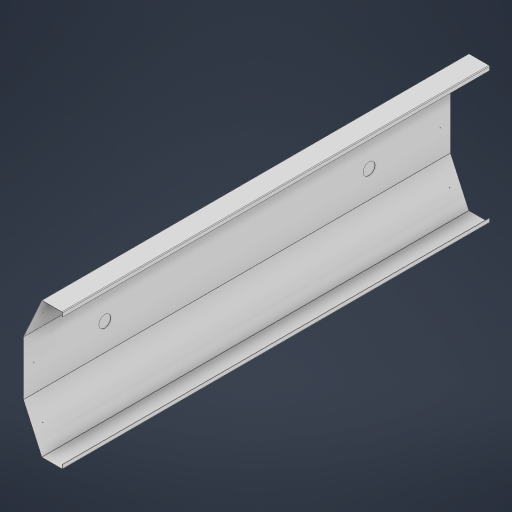
# Autodesk Inventor part: Carcasa
Saved by Autodesk Inventor 2024 (Build 280153000, 153)
## iProperties
Created: 2023-04-23
Part Number: Carcasa
Material: Genérico
Document SubType Name: Sheet Metal
Designer: javie
Density: 1 g/cm^3
Sheet Metal Rule: Por defecto_mm
Appearance: Valor por defecto
Author: javie
Autodesk Inventor part; units mm, degrees
note: some values were not read from the file. Chosen so that the rebuilt part matches the saved one: flange form of "Placa1".
ref_plane "YZ Plane" through (0, 0, 0) normal (1, 0, 0) x (0, 1, 0)
ref_plane "XZ Plane" through (0, 0, 0) normal (0, 1, 0) x (-1, 0, 0)
ref_plane "XY Plane" through (0, 0, 0) normal (0, 0, 1) x (1, 0, 0)
sketch "Boceto1" plane through (0, 0, 0) normal (0, 0, 1) x (1, 0, 0)
  line L0 (-10, 6.5506) -> (-10, 58.1012)
  line L1 (-10, 58.1012) -> (17.1565, 118.1012)
  line L2 (17.1565, 118.1012) -> (47.1565, 118.1012)
  line L3 (47.1565, 118.1012) -> (47.1565, 112.4113)
  line L4 (-10, 6.5506) -> (-10, -21.8988)
  line L5 (-10, -21.8988) -> (17.1565, -81.8988)
  line L6 (17.1565, -81.8988) -> (47.1565, -81.8988)
  line L7 (47.1565, -81.8988) -> (47.1565, -76.2089)
  point P0 (47.1565, 115.2562)
  dimension "d22" = 60
  dimension "d23" = 60
  dimension "d24" = 30
  dimension "d25" = 30
  dimension "d26" = 200
  dimension "d44" = 57.1565
  measures "d22" vertical distance of L0.end L1.end
  measures "d23" vertical distance of L5.start L6.start
  measures "d24" distance of L1.end L2.end
  measures "d25" distance of L6.start L7.start
  measures "d26" distance of L7.start L2.end
  measures "d44" distance from line of L0 point (47.156, 115.256)
contour flange "Pestaña de contorno1" sketch "Boceto1" thickness 0.5 bend radius 0.5 width 629.96 along (0, 0, 1) mid plane no both sides no wall seen from (47.1565, 115.2562, 0) lies toward (1, 0, 0) curves L3 L2 L1 L0 L4 L5 L6 L7
bend "Doblez1"
corner "Esquina1"
sketch "Boceto2" plane through (-10, -21.7909, 629.96) normal (1, 0, 0) x (0, 0, -1)
  circle A0 centre (614.96, 39.8921) radius 0.5
  line L0 (629.96, 79.7842) -> (629.96, 0) projected
  circle A1 centre (15, 39.8921) radius 0.5
  line L1 (0, 0) -> (0, 79.7842) projected
  circle A2 centre (120, 39.8921) radius 9
  circle A3 centre (509.96, 39.8921) radius 9
  point P0 (629.96, 21.7909)
  point P1 (0, 39.8921)
  point P2 (629.96, 39.8921)
  dimension "d16" = 1
  dimension "d17" = 15
  dimension "d18" = 1
  dimension "d19" = 15
  dimension "d27" = 0
  dimension "d40" = 18
  dimension "d41" = 18
  dimension "d42" = 120
  dimension "d43" = 120
  constraints: 4 centre point, 2 midpoint
  measures "d16" diameter of A0
  measures "d17" distance from line of L0 A0.centre
  measures "d18" diameter of A1
  measures "d19" distance of point (0, 39.892) A1.centre
  measures "d27" vertical distance of point (629.96, 39.892) A0.centre
  measures "d40" diameter of A2
  measures "d41" diameter of A3
  measures "d42" distance from line of L1 A2.centre
  measures "d43" distance from line of L0 A3.centre
extrude "Extrusión1" cut sketch "Boceto2" against normal blind 10
sketch "Boceto3" plane through (-9.9555, 58.1995, 629.96) normal (0.9110302, -0.4123397, 0) x (0, 0, -1)
  circle A0 centre (15, 32.7145) radius 0.5
  line L0 (0, 0) -> (0, 65.4291) projected
  circle A1 centre (614.96, 32.7145) radius 0.5
  line L1 (629.96, 65.4291) -> (629.96, 0) projected
  point P0 (629.96, -48.9164)
  dimension "d28" = 1
  dimension "d29" = 15
  dimension "d30" = 1
  dimension "d31" = 15
  constraints: 2 centre point
  measures "d28" diameter of A0
  measures "d29" distance from line of L0 A0.centre
  measures "d30" diameter of A1
  measures "d31" distance from line of L1 A1.centre
extrude "Extrusión2" cut sketch "Boceto3" against normal blind 4.25
sketch "Boceto4" plane through (17.0235, -81.605, 629.96) normal (0.9110302, 0.4123397, 0) x (0, 0, -1)
  circle A0 centre (15, 32.7145) radius 0.5
  line L0 (0, 0) -> (0, 65.4291) projected
  circle A1 centre (614.96, 32.7145) radius 0.5
  line L1 (629.96, 65.4291) -> (629.96, 0) projected
  point P0 (629.96, 81.3641)
  point P1 (0, 32.7145)
  dimension "d34" = 1
  dimension "d35" = 15
  dimension "d36" = 1
  dimension "d37" = 15
  constraints: 2 centre point, 1 midpoint
  measures "d34" diameter of A0
  measures "d35" distance of point (0, 32.715) A0.centre
  measures "d36" diameter of A1
  measures "d37" distance from line of L1 A1.centre
extrude "Extrusión3" cut sketch "Boceto4" against normal blind 6
sketch "Boceto6" plane through (-10.5, -21.7909, 0) normal (-1, 0, 0) x (0, 0, 1)
  circle A0 centre (120, 39.8921) radius 9 projected
  circle A1 centre (120, 39.8921) radius 9
  circle A2 centre (509.96, 39.8921) radius 9 projected
  circle A3 centre (509.96, 39.8921) radius 9
  point P0 (0, 21.7909)
  constraints: 2 centre point, 2 coincident
extrude "Extrusión4" add sketch "Boceto6" along normal blind 1
equation "\"d5\" = Grosor"
equation "\"d6\" = Anchura_desahogo_plegado"
equation "\"d7\" = Profundidad_desahogo_plegado"
equation "\"d8\" = Remanente_mínimo"
equation "\"d9\" = Radiodetransición"
equation "\"d11\" = Radio_pliegue"
equation "\"d13\" = Tamaño_destalonado"
equation "\"d14\" = TamañoSeparación"
equation "\"d15\" = Tamaño_de_radio_de_Jacobi"
equation "\"Radio_pliegue\" = Grosor"
equation "\"Remanente_mínimo\" = 2 * Grosor"
equation "\"TamañoSeparación\" = Grosor"
equation "\"Radiodetransición\" = Radio_pliegue"
equation "\"Tamaño_destalonado\" = 4 * Grosor"
equation "\"Anchura_desahogo_plegado\" = Grosor"
equation "\"Tamaño_de_radio_de_Jacobi\" = Radio_pliegue"
equation "\"Profundidad_desahogo_plegado\" = 0.5 * Grosor"
equation "\"Grosor\" = 0.5"
